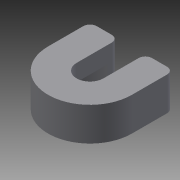
# Autodesk Inventor part: HeadConnector
Saved by Autodesk Inventor 2014 SP1 (Build 180222100, 222)
## iProperties
Created: 2013-10-30
Part Number: HeadConnector
Material: Generic
Document SubType Name: Modeling
Designer: david
Density: 1 g/cm^3
Appearance: Default
HeadConnectorDiam: 12,000 mm
HeadConnectorHeight: 3,000 mm
HeadConnectorOuterSize: 15,000 mm
HeadConnectorWidth: 4,800 mm
HeadConnectorOuterHeight: 3,000 mm
HeadConnectorTolerance: 0,200 mm
HeadConnectorProportion: 0,600 ul
Author: david
Autodesk Inventor part; units mm, degrees
ref_plane "YZ Plane" through (0, 0, 0) normal (1, 0, 0) x (0, 1, 0)
ref_plane "XZ Plane" through (0, 0, 0) normal (0, 1, 0) x (-1, 0, 0)
ref_plane "XY Plane" through (0, 0, 0) normal (0, 0, 1) x (1, 0, 0)
sketch "Sketch1" plane through (0, 0, 0) normal (0, 1, 0) x (-1, 0, 0)
  arc A0 (7.5, 0) -> (-7.5, 0) centre (0, 0) ccw
  arc A1 (2.4, 0) -> (-2.4, 0) centre (0, 0) ccw
  line L0 (-7.5, 0) -> (7.5, 0) construction
  line L1 (0, 0) -> (0, 11.6178) construction
  line L2 (-7.5, 0) -> (-7.5, -7.5)
  line L3 (-2.4, 0) -> (-2.4, -7.5)
  line L4 (2.4, 0) -> (2.4, -7.5)
  line L5 (7.5, 0) -> (7.5, -7.5)
  line L6 (-7.5, -7.5) -> (-2.4, -7.5)
  line L7 (2.4, -7.5) -> (7.5, -7.5)
  dimension "d0" = 15
  dimension "d2" = 7.5
  dimension "d3" = 4.8
  dimension "d6" = 7.5
  dimension "d8" = 7.5
  constraints: 16 end point, 4 point on circle, 4 tangent, 3 parallel, 2 centre point, 2 coincident, 2 point on line, 1 horizontal, 1 perpendicular
  measures "d0" distance of L0.end L0.start
  measures "d2" radius of A0
  measures "d3" distance of L3.start L4.start
  measures "d6" distance of L2.end L0.start
  measures "d8" distance from line of L1.end L5
extrude "Extrusion1" add sketch "Sketch1" against normal blind 3
sketch "Sketch2" plane through (0, -3, 0) normal (0, -1, 0) x (1, 0, 0)
  arc A0 (7.5, 0) -> (-7.5, 0) centre (0, 0) ccw projected
  line L0 (-7.5, 0) -> (-7.5, -7.5) projected
  line L1 (-2.4, -7.5) -> (-2.4, 0) projected
  arc A1 (2.4, 0) -> (-2.4, 0) centre (0, 0) ccw projected
  line L2 (2.4, 0) -> (2.4, -7.5) projected
  line L3 (7.5, -7.5) -> (7.5, 0) projected
  arc A2 (2.4, -5.4991) -> (-2.4, -5.4991) centre (0, 0) ccw
  arc A3 (7.5, 0) -> (-7.5, 0) centre (0, 0) ccw
  line L4 (-7.5, 0) -> (-7.5, -7.5)
  line L5 (-2.4, -7.5) -> (-2.4, -5.4991)
  line L6 (2.4, -5.4991) -> (2.4, -7.5)
  line L7 (7.5, -7.5) -> (7.5, 0)
  line L8 (-7.5, -7.5) -> (-2.4, -7.5)
  line L9 (2.4, -7.5) -> (7.5, -7.5)
  dimension "d11" = 6
  constraints: 12 end point, 5 point on circle, 4 tangent, 3 collinear, 2 centre point, 2 coincident, 2 point on line, 1 parallel, 1 perpendicular
  measures "d11" radius of A2
extrude "Extrusion2" add sketch "Sketch2" along normal blind 3 contours L3 L9 L2 A2 L1 L8 L0 A0
fillet "Fillet1" radius 1.2 1 edges at (7.5, -3, -7.5)
fillet "Fillet2" radius 1.2 3 edges at (2.4, -3, -7.5) (-2.4, -3, -7.5) (-7.5, -3, -7.5)
sketch "Sketch3" plane through (0, -3, 0) normal (0, -1, 0) x (1, 0, 0)
  arc A0 (2.4, -5.4991) -> (-2.4, -5.4991) centre (0, 0) ccw projected
  line L0 (-2.4, -5.4991) -> (-2.4, 0) projected
  arc A1 (2.4, 0) -> (-2.4, 0) centre (0, 0) ccw projected
  line L1 (2.4, 0) -> (2.4, -5.4991) projected
  line L2 (0, 13.9059) -> (0, -15.9339) construction
  line L3 (-15.9969, 0.3837) -> (17.7517, -5.5671) construction
  line L4 (-15.1634, 5.1107) -> (18.5852, -0.84) construction
  line L5 (-2.4, -15.573) -> (-2.4, 20.0388) construction
  line L6 (2.4, -5.4991) -> (2.4, -2.8602)
  line L7 (4.9988, -3.3184) -> (2.4, -2.8602)
  line L8 (-4.9988, 3.3184) -> (-2.4, 2.8602)
  line L9 (-2.4, 5.4991) -> (-2.4, 2.8602)
  arc A2 (-3, 5.1962) -> (-4.9988, 3.3184) centre (0, 0) ccw
  arc A3 (2.4, -5.4991) -> (4.9988, -3.3184) centre (0, 0) ccw
  dimension "d27" = 80
  constraints: 16 end point, 7 point on circle, 7 point on line, 3 collinear, 3 parallel, 2 centre point, 2 coincident, 2 tangent
  measures "d27" angle of L2 L4
extrude "Extrusion3" add sketch "Sketch3" along normal blind 3 contours L1 L7 A0 | L9 L8 A0
equation "\"d0\" = HeadConnectorOuterSize"
equation "\"d2\" = 0.5 * HeadConnectorOuterSize"
equation "\"d3\" = HeadConnectorWidth"
equation "\"d6\" = 0.5 * HeadConnectorOuterSize"
equation "\"d8\" = 0.5 * HeadConnectorOuterSize"
equation "\"d9\" = HeadConnectorOuterHeight"
equation "\"d11\" = 0.5 * HeadConnectorDiam"
equation "\"d12\" = HeadConnectorHeight"
equation "\"d14\" = 2 * HeadConnectorProportion"
equation "\"d15\" = 2 * HeadConnectorProportion"
equation "\"d28\" = HeadConnectorHeight"
equation "\"HeadConnectorDiam\" = 20 * HeadConnectorProportion"
equation "\"HeadConnectorWidth\" = 8 * HeadConnectorProportion"
equation "\"HeadConnectorOuterSize\" = 25 * HeadConnectorProportion"
equation "\"HeadConnectorHeight\" = 5 * HeadConnectorProportion"
equation "\"HeadConnectorOuterHeight\" = 5 * HeadConnectorProportion"
equation "\"HeadConnectorTolerance\" = 0.2"
equation "\"HeadConnectorProportion\" = 0.6"
body "Solid1"
